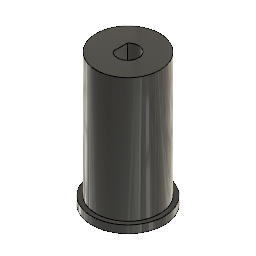
omniwheel_adapter (Autodesk Fusion 360 design; units mm, degrees)
Autodesk Fusion 360 part; units mm, degrees
sketch "Sketch1" plane through (0, 0, 0) normal (0, 0, 1) x (1, 0, 0)
  circle A0 centre (0, 0) radius 7
  circle A1 centre (0, 0) radius 6.15
  circle A2 centre (0, 0) radius 2.05
  line L0 (-1.5, 0) -> (-1.5, -1.3973)
  line L1 (-1.5, 0) -> (-1.5, 1.3973)
  point P0 (-1.5, 0)
  dimension "d1" = 14
  dimension "d2" = 12.3
  dimension "d3" = 4.1
  dimension "d4" = 1.5
  constraint coincident A0.centre A1.centre
  constraint concentric A0 A1
  constraint coincident A2 L0.end
  constraint coincident P0 L0.start
  constraint vertical L0
  constraint coincident A2 L1.end
  constraint parallel L0 L1
  measures "d1" diameter of A0
  measures "d2" diameter of A1
  measures "d3" diameter of A2
  measures "d4" distance of A0.centre P0
extrude "Extrude1" add sketch "Sketch1" along normal blind 1.5 contours A0 | A1 | A2 L0 L1 | A2 L0 L1
extrude "Extrude2" add sketch "Sketch1" along normal blind 25.5 contours A1 | A2 L0 L1 picked at (-1.859, 0.1021)
extrude "Extrude3" add sketch "Sketch1" along normal blind 7.5 contours A2 L0 L1 picked at (0.859, -0.1018)
